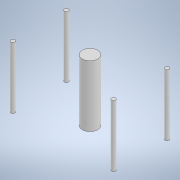
# Autodesk Inventor part: Joystick_Holes_Positive
Saved by Autodesk Inventor 2022 (Build 260153000, 153)
## iProperties
Created: 2023-04-12
Part Number: Joystick_Holes_Positive
Material: Generic
Document SubType Name: Modeling
Designer: Staff
Density: 1 g/cm^3
Appearance: Default
Author: Staff
Autodesk Inventor part; units mm, degrees
ref_plane "YZ Plane" through (0, 0, 0) normal (1, 0, 0) x (0, 1, 0)
ref_plane "XZ Plane" through (0, 0, 0) normal (0, 1, 0) x (-1, 0, 0)
ref_plane "XY Plane" through (0, 0, 0) normal (0, 0, 1) x (1, 0, 0)
sketch "Sketch1" plane through (0, 0, 0) normal (0, 1, 0) x (-1, 0, 0)
  line L0 (41.04, -21.775) -> (-41.04, -21.775) construction
  line L1 (-41.04, -21.775) -> (-41.04, 21.775) construction
  line L2 (-41.04, 21.775) -> (41.04, 21.775) construction
  line L3 (41.04, 21.775) -> (41.04, -21.775) construction
  circle A0 centre (-41.04, -21.775) radius 1.65
  circle A1 centre (-41.04, 21.775) radius 1.65
  circle A2 centre (41.04, 21.775) radius 1.65
  circle A3 centre (41.04, -21.775) radius 1.65
  circle A4 centre (0, 0) radius 6.25
  line L4 (41.04, -21.775) -> (-41.04, -21.775) construction
  line L5 (-41.04, -21.775) -> (-41.04, 21.775) construction
  line L6 (-41.04, 21.775) -> (41.04, 21.775) construction
  line L7 (41.04, 21.775) -> (41.04, -21.775) construction
  line L8 (41.04, -21.775) -> (-41.04, 21.775) construction
  line L9 (-41.04, -21.775) -> (41.04, 21.775) construction
  circle A5 centre (41.04, -78.2405) radius 1.65 construction
  line L10 (41.04, -78.2405) -> (41.04, -21.775) construction
  point P0 (0, 0)
  dimension "d0" = 82.08
  dimension "d1" = 43.55
  dimension "d2" = 3.3
  dimension "d3" = 12.5
  dimension "d6" = 56.4655
  dimension "d7" = 41.04
  constraints: 22 end point, 6 centre point, 5 coincident, 4 midpoint, 4 parallel, 3 equal radius, 2 horizontal, 2 horizontal alignment, 2 perpendicular, 1 vertical, 1 vertical alignment
  measures "d0" distance of L0.start L1.start
  measures "d1" distance of L3.start L0.start
  measures "d2" diameter of A3
  measures "d3" diameter of A4
  measures "d6" distance of A5.centre L10.end
  measures "d7" horizontal distance of point (0, 0) A5.centre
extrude "Extrusion1" add sketch "Sketch1" along normal mid plane 50
body "Solid1"
